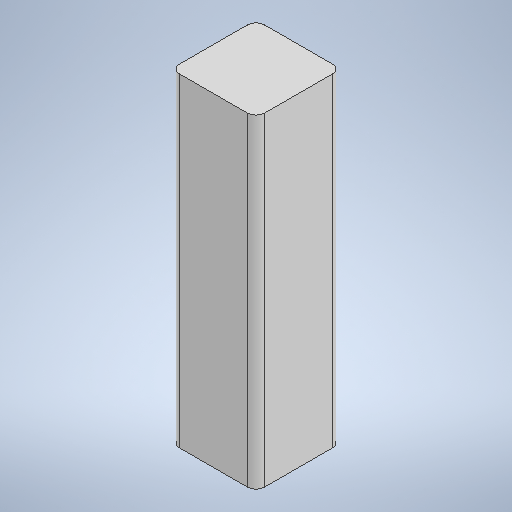
# Autodesk Inventor part: Item4040BearingHolder
Saved by Autodesk Inventor 2025.1 (Build 291241000, 241)
## iProperties
Created: 2025-10-12
Part Number: Item4040BearingHolder
Material: Generic
Document SubType Name: Modeling
Designer: jonas
Density: 1 g/cm^3
Appearance: Default
Author: jonas
Autodesk Inventor part; units mm, degrees
ref_plane "YZ Plane" through (0, 0, 0) normal (1, 0, 0) x (0, 1, 0)
ref_plane "XZ Plane" through (0, 0, 0) normal (0, 1, 0) x (-1, 0, 0)
ref_plane "XY Plane" through (0, 0, 0) normal (0, 0, 1) x (1, 0, 0)
sketch "Sketch1" plane through (0, 0, 0) normal (0, 1, 0) x (-1, 0, 0)
  line L0 (0, -18.0149) -> (0, 18.0149) construction
  line L1 (12.8536, 0) -> (-12.8536, 0) construction
  line L2 (16, -20) -> (-16, -20)
  arc A0 (16, -20) -> (20, -16) centre (16, -16) ccw
  line L3 (20, 16) -> (20, -16)
  arc A1 (20, 16) -> (16, 20) centre (16, 16) ccw
  line L4 (-16, 20) -> (16, 20)
  arc A2 (-20, -16) -> (-16, -20) centre (-16, -16) ccw
  arc A3 (-16, 20) -> (-20, 16) centre (-16, 16) ccw
  line L5 (-20, -16) -> (-20, 16)
  point P0 (0, 0)
  point P1 (0, 0)
  point P2 (0, 0)
  point P3 (0, 0)
  point P4 (-20, -20)
  point P5 (20, -20)
  point P6 (20, 20)
  point P7 (-20, 20)
  dimension "d0" = 40
  dimension "d1" = 40
  dimension "d2" = 4
  constraints: 12 end point, 8 point on circle, 8 point on line, 8 tangent, 4 centre point, 3 coincident, 3 equal radius, 2 horizontal, 2 midpoint, 2 parallel, 1 perpendicular, 1 vertical, 2 other
  measures "d0" distance between parallel lines of L4 L2
  measures "d1" distance between parallel lines of L3 L5
  measures "d2" radius of A3
extrude "Extrusion1" add sketch "Sketch1" along normal blind 152.5
body "Solid1"
